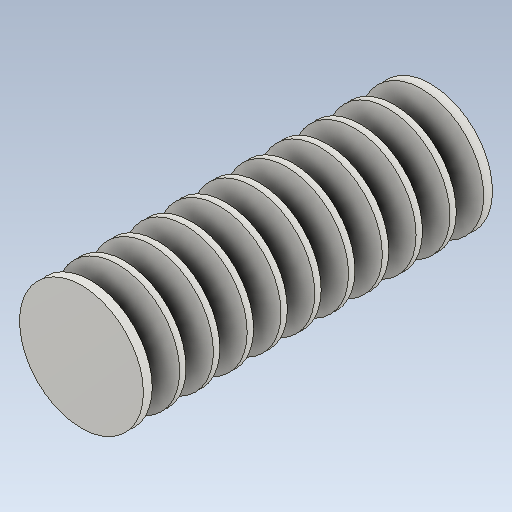
# Autodesk Inventor part: Grooved Pulley1
Saved by Autodesk Inventor 2021.1 (Build 251245000, 245)
## iProperties
Created: 2021-01-01
Part Number: Grooved Pulley1
Material: Steel
Document SubType Name: Modeling
Designer: Bolisteward
Density: 1 g/cm^3
Appearance: Steel
CustomPartVersion: 1
Author: Bolisteward
Autodesk Inventor part; units mm, degrees
ref_plane "YZ Plane" through (0, 0, 0) normal (1, 0, 0) x (0, 1, 0)
ref_plane "XZ Plane" through (0, 0, 0) normal (0, 1, 0) x (-1, 0, 0)
sketch "Main Sketch" plane through (0, 0, 0) normal (1, 0, 0) x (0, 1, 0)
  line L0 (0, 124) -> (22, 124)
  line L1 (22, 124) -> (22, 12.8615)
  line L2 (22, 12.8615) -> (11, 9.4984)
  line L3 (11, 9.4984) -> (11, 6.5016)
  line L4 (11, 6.5016) -> (22, 3.1385)
  line L5 (22, 3.1385) -> (22, 0)
  line L6 (22, 0) -> (0, 0)
  line L7 (20, 12.25) -> (20, 3.75) construction
  line L8 (11, 8) -> (20, 8) construction
  line L9 (22, 12.8615) -> (22, 3.1385)
  line L10 (0, -4) -> (0, 24) projected
  line L11 (0, 0) -> (0, 124)
  dimension "d0" = 8.5
  dimension "d1" = 34
  dimension "d2" = 2
  dimension "d6" = 124
  dimension "d21" = 40
  dimension "d25" = 11
  dimension "d27" = 8
  constraints: 22 end point, 5 perpendicular, 2 collinear, 2 midpoint, 2 point on line, 1 parallel
  measures "d0" distance of L7.start L7.end
  measures "d1" angle of L2 L4
  measures "d2" distance between parallel lines of L1 L7
  measures "d6" distance between parallel lines of L6 L0
  measures "d21" diameter of L7 L10
  measures "d25" distance between parallel lines of L3 L9
  measures "d27" distance between parallel lines of L6 L8
ref_plane "Belt Plane" through (0, 11, 8) normal (0, 0, 1) x (1, 0, 0)
revolve "Body" add sketch "Main Sketch" angle 360 about axis through (0, 0, -10) along (0, 0, 1)
revolve "Groove" cut sketch "Main Sketch" angle 360 about axis through (0, 0, -10) along (0, 0, 1) contours L9 L4 L3 L2
fillet "Fillet External" [suppressed]
fillet "Fillet Internal" [suppressed]
pattern_linear "Groove Pattern" count 10 spacing 12 along (0, 0, 1) of "Groove"
equation "\"d0\" = da_Bw"
equation "\"d1\" = da_Alfa"
equation "\"d2\" = da_c"
equation "\"d21\" = da_Dw"
equation "\"d25\" = da_Hd"
equation "\"d27\" = da_Se"
equation "\"da_r1\" = 0"
equation "\"da_r2\" = 0"
equation "\"d18\" = da_Sg"
equation "\"d5\" = da_Se"
equation "\"da_Bw\" = 8.5"
equation "\"da_Alfa\" = 34deg"
equation "\"da_c\" = 2"
equation "\"da_Dw\" = 40"
equation "\"da_Hd\" = 11"
equation "\"da_Se\" = 8"
equation "\"da_Sg\" = 12"
body "Solid1"
